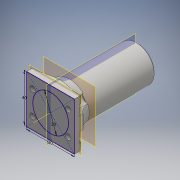
# Autodesk Inventor part: arbre_central_4040_rev10
Saved by Autodesk Inventor 2016 (Build 200138000, 138)
## iProperties
Created: 2018-04-11
Part Number: arbre_central_4040_rev10
Material: Generic
Document SubType Name: Modeling
Designer: mbouhier
Density: 1 g/cm^3
Appearance: Default
Author: mbouhier
Autodesk Inventor part; units mm, degrees
ref_plane "YZ Plane" through (0, 0, 0) normal (1, 0, 0) x (0, 1, 0)
ref_plane "XZ Plane" through (0, 0, 0) normal (0, 1, 0) x (-1, 0, 0)
ref_plane "XY Plane" through (0, 0, 0) normal (0, 0, 1) x (1, 0, 0)
sketch "Sketch1" plane through (0, 0, 0) normal (0, 1, 0) x (-1, 0, 0)
  line L0 (-20, 20) -> (20, 20)
  line L1 (20, 20) -> (20, -20)
  line L2 (20, -20) -> (-20, -20)
  line L3 (-20, -20) -> (-20, 20)
  line L4 (-20, 20) -> (20, -20) construction
  line L5 (20, 20) -> (-20, -20) construction
  circle A0 centre (0, 0) radius 15
  dimension "d0" = 40
  dimension "d1" = 40
  dimension "d2" = 30
  constraints: 12 end point, 2 midpoint, 2 parallel, 1 centre point, 1 coincident, 1 horizontal, 1 perpendicular
  measures "d0" distance of L1.end L2.end
  measures "d1" distance of L0.end L1.end
  measures "d2" diameter of A0
extrude "Extrusion1" add sketch "Sketch1" along normal blind 73 contours A0
extrude "Extrusion2" add sketch "Sketch1" along normal blind 5
ref_plane "Work Plane1" through (0, 16, 0) normal (0, -1, 0) x (1, 0, 0)
sketch "Sketch2" plane through (0, 16, 0) normal (0, -1, 0) x (1, 0, 0)
  circle A0 centre (0, 0) radius 16.5
  circle A1 centre (0, 0) radius 15 projected
  dimension "d8" = 33
  constraints: 1 centre point, 1 coincident
  measures "d8" diameter of A0
extrude "Extrusion3" add sketch "Sketch2" along normal up to next
fillet "Fillet1" radius 11 1 edges at (-16.5, 5, 0)
ref_plane "Work Plane2" through (0, 4, 0) normal (0, -1, 0) x (1, 0, 0)
sketch "Sketch3" plane through (0, 4, 0) normal (0, -1, 0) x (1, 0, 0)
  line L0 (20, 20) -> (-20, 20) projected
  line L1 (-20, 20) -> (-20, -20) projected
  line L2 (-20, -20) -> (20, -20) projected
  line L3 (20, -20) -> (20, 20) projected
  circle A0 centre (-15, -10) radius 2.25
  circle A1 centre (-15, 10) radius 2.25
  arc A2 (-15, -14) -> (-15, -6) centre (-15, -10) ccw
  arc A3 (-15, 6) -> (-15, 14) centre (-15, 10) ccw
  line L4 (-15, -14) -> (-20, -14)
  line L5 (-20, 20) -> (-20, -20) projected
  line L6 (-15, -6) -> (-20, -6)
  line L7 (-15, 6) -> (-20, 6)
  line L8 (-15, 14) -> (-20, 14)
  line L9 (-20, -14) -> (-20, -6)
  line L10 (-20, 6) -> (-20, 14)
  point P0 (0, 0)
  dimension "d13" = 5
  dimension "d14" = 10
  dimension "d15" = 10
  dimension "d17" = 4.5
  dimension "d20" = 8
  dimension "d21" = 8
  constraints: 12 end point, 4 centre point, 4 coincident, 4 point on circle, 4 point on line, 3 parallel, 2 collinear, 1 perpendicular
  measures "d13" distance from line of L1 point (-15, -10)
  measures "d14" distance from line of L2 point (-15, -10)
  measures "d15" distance from line of point (-15, 10) L0
  measures "d17" diameter of A0
  measures "d20" diameter of A2
  measures "d21" diameter of A3
extrude "Extrusion4" cut sketch "Sketch3" against normal up to surface (12 mm away) contours L8 A3 L7 L1 | L1 L6 A2 L4 | A0 | A1
extrude "Extrusion5" cut sketch "Sketch3" along normal blind 10 contours A0 | A1
ref_plane "Work Plane3" through (0, 0, -20) normal (-1, 0, 0) x (0, 0, 1)
mirror "Mirror1" about plane through (0, 0, -20) normal (-1, 0, 0) of "Extrusion4", "Extrusion5"
sketch "Sketch4" plane through (0, 73, 0) normal (0, 1, 0) x (1, 0, 0)
  circle A0 centre (0, 0) radius 11
  point P0 (-11, 0)
  dimension "d28" = 22
  constraints: 1 coincident, 1 horizontal alignment, 2 other
hole "Hole1" at (-11, 73, 0) direction (0, -1, 0) diameter 4 depth 6
pattern_circular "Circular Pattern1" count 3 over 360 about axis through (0, -10, 0) along (0, 1, 0) of "Hole1"
chamfer "Chamfer1" distance 1 angle 45 1 edges at (15, 73, 0)
sketch "Sketch5" plane through (20, 0, -20) normal (0, 0, -1) x (-1, 0, 0)
  line L0 (19.5132, 8.5076) -> (20.5132, 8.5076)
  line L1 (20.5132, 8.5076) -> (20.5132, -0.4924)
  line L2 (20.5132, -0.4924) -> (19.5132, -0.4924)
  line L3 (19.5132, -0.4924) -> (19.5132, 8.5076)
  line L4 (19.5132, 8.5076) -> (20.5132, -0.4924) construction
  line L5 (20.5132, 8.5076) -> (19.5132, -0.4924) construction
  point P0 (20, 0)
  point P1 (20.0132, 4.0076)
  point P2 (20.0132, 4.0076)
  dimension "d42" = 1
  dimension "d43" = 9
  constraints: 12 end point, 2 midpoint, 2 parallel, 1 coincident, 1 horizontal, 1 perpendicular
  measures "d42" distance of L1.end L2.end
  measures "d43" distance of L0.end L1.end
extrude "Extrusion6" cut sketch "Sketch5" against normal blind 1
equation "\"d15\" = d14"
equation "\"d21\" = d20"
body "Solid1"
